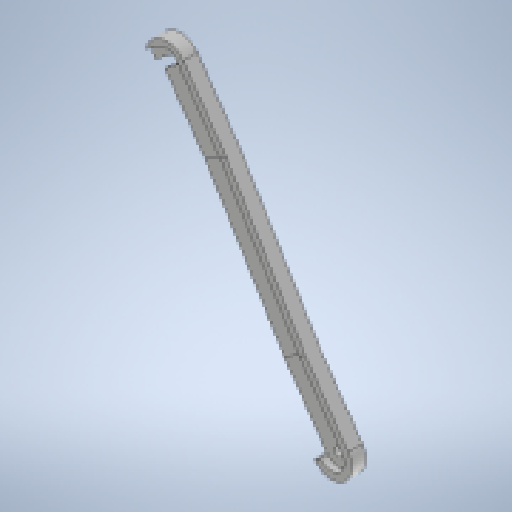
# Autodesk Inventor part: TheHandle_LeftBack
Saved by Autodesk Inventor 2025.1 (Build 291241000, 241)
## iProperties
Created: 2026-05-10
Part Number: TheHandle_LeftBack
Material: Generic
Document SubType Name: Modeling
Designer: User
Density: 1 g/cm^3
Appearance: Default
Author: User
## iProperties of the stored document TheHandle_LeftBack_3DPrint.ipt
Created: 2026-05-12
Part Number: TheHandle_LeftBack_3DPrint
Material: Generic
Document SubType Name: Modeling
Designer: User
Density: 1 g/cm^3
Appearance: Default
Author: User
Autodesk Inventor part; units mm, degrees
ref_plane "YZ Plane" through (0, 0, 0) normal (1, 0, 0) x (0, 1, 0)
ref_plane "XZ Plane" through (0, 0, 0) normal (0, 1, 0) x (-1, 0, 0)
ref_plane "XY Plane" through (0, 0, 0) normal (0, 0, 1) x (1, 0, 0)
sketch "Sketch1" plane through (0, 0, 0) normal (0, 0, 1) x (1, 0, 0)
  arc A0 (17.8, -18.3349) -> (28.2, -18.3349) centre (23, -18.3349) ccw projected
  circle A1 centre (120.0032, -158.8554) radius 2.5 projected
  arc A2 (212.7339, -15.835) -> (209.4702, -20.8697) centre (211.0753, -18.3349) ccw projected
  circle A3 centre (23, -18.3349) radius 2.5
  circle A4 centre (23, -18.3349) radius 7.5
  circle A5 centre (120.0032, -158.8554) radius 7.5
  line L0 (113.831, -163.1162) -> (16.8278, -22.5957)
  line L1 (126.1754, -154.5947) -> (29.1722, -14.0742)
  point P0 (0, 0)
  dimension "d0" = 5
  dimension "d1" = 15
  dimension "d2" = 15
  constraints: 4 end point, 4 point on circle, 4 tangent, 3 centre point, 3 coincident
  measures "d0" diameter of A3
  measures "d1" diameter of A4
  measures "d2" diameter of A5
extrude "Extrusion1" add sketch "Sketch1" along normal blind 4
sketch "Sketch2" plane through (113.831, -163.1162, 0) normal (-0.8229595, -0.5681, 0) x (0, 0, 1)
  line L0 (4, 170.7502) -> (4, 0) projected
  line L1 (8, 170.7502) -> (8, 0)
  line L2 (8, 85.3751) -> (0, 85.3751)
  line L3 (0, 170.7502) -> (0, 0) projected
  line L4 (8, 0) -> (8, 85.3751)
  line L5 (8, 42.6875) -> (0, 42.6875)
  line L6 (8, 170.7502) -> (8, 85.3751)
  line L7 (8, 128.0626) -> (0, 128.0626)
  line L8 (4, 42.6875) -> (0, 128.0626)
  line L9 (8, 42.6875) -> (4, 128.0626)
  line L10 (8, 0) -> (4, 0)
  point P0 (0, 198.9054)
  dimension "d5" = 4
  constraints: 18 end point, 6 midpoint, 3 perpendicular, 2 collinear, 2 point on line, 1 parallel
  measures "d5" distance between parallel lines of L0 L1
extrude "Extrusion2" add sketch "Sketch2" against normal up to surface (15 mm away) contours L5 L1 L10 L0 | L0 L2 L9 L5 | L0 L9 L2
sketch "Sketch3" plane through (16.8278, -22.5957, 0) normal (-0.8229595, -0.5681, 0) x (0, 0, 1)
  line L0 (0, 0) -> (0, -170.7502) projected
  line L1 (0, -170.7502) -> (4, -170.7502) projected
  line L2 (4, -170.7502) -> (8, -170.7502) projected
  line L3 (8, -170.7502) -> (8, -128.0626) projected
  line L4 (8, -128.0626) -> (4, -42.6875) projected
  line L5 (4, 0) -> (4, -42.6875) projected
  line L6 (0, 0) -> (4, 0) projected
  line L7 (4, -170.7502) -> (4, -173.2502) projected
  line L8 (4, -170.7502) -> (4, -42.6875)
  line L9 (0, -170.7502) -> (0, 0) projected
  line L10 (8, -170.7502) -> (8, -128.0626) projected
  line L11 (8, -128.0626) -> (4, -128.0626)
  line L12 (4, -128.0626) -> (0, -42.6875)
  line L13 (0, -178.2502) -> (4, -178.2502)
  line L14 (4, -166.4894) -> (4, -164.4356) projected
  line L15 (0, -178.2502) -> (0, -163.8178) projected
  point P0 (0, 28.1552)
  constraints: 6 end point, 2 parallel, 2 point on line, 1 perpendicular, 5 other
extrude "Extrusion3" cut sketch "Sketch3" against normal through all contours L12 L8 L1 L0 | L8 L4 L11
sketch "Sketch4" plane through (113.831, -163.1162, 8) normal (0, 0, 1) x (0.8229595, 0.5681, 0)
  circle A0 centre (7.5, 0) radius 2.5 projected
  arc A1 (3.4533, 6.3146) -> (1.3278, 4.2607) centre (7.5, 0) ccw projected
  circle A2 centre (7.5, 0) radius 2.5
  point P0 (-1.012, 198.9054)
  constraints: 1 centre point, 1 coincident, 1 concentric
extrude "Extrusion4" cut sketch "Sketch4" against normal blind 10
sketch "Sketch5" plane through (113.831, -163.1162, 8) normal (0, 0, 1) x (0.8229595, 0.5681, 0)
  circle A0 centre (7.5, 0) radius 2.5 projected
  line L0 (15, 0) -> (15, 42.6875) projected
  line L1 (0, 0) -> (0, 42.6875) projected
  line L2 (10, 0) -> (15, 0) projected
  circle A1 centre (7.5, 0) radius 7.5
  point P0 (-1.012, 198.9054)
  constraints: 2 horizontal alignment, 1 coincident, 2 other
extrude "Extrusion5" add sketch "Sketch5" against normal blind 4
sketch "Sketch6" plane through (0, 0, 4) normal (0, 0, 1) x (1, 0, 0)
  circle A0 centre (23, -18.3349) radius 2.5 projected
  line L0 (53.423, -49.2043) -> (29.1722, -14.0742) projected
  arc A1 (18.7282, -24.4995) -> (16.8278, -22.5957) centre (23, -18.3349) ccw
  circle A2 centre (120.0032, -158.8554) radius 2.5 projected
  arc A3 (24.4203, -20.3923) -> (18.3431, -24.7907) centre (120.0032, -158.8554) ccw
  arc A4 (21.5797, -16.2775) -> (15.8025, -20.4436) centre (120.0032, -158.8554) ccw
  line L1 (16.8278, -22.5957) -> (41.0786, -57.7258) projected
  point P0 (0, 0)
  dimension "d14" = 5
  constraints: 11 point on circle, 3 centre point, 2 coincident, 1 end point, 1 point on line, 1 tangent
  measures "d14" radial gap between concentric circles of A3 A4
extrude "Extrusion6" cut sketch "Sketch6" against normal blind 4 contours A0 A3 L1 A1 A4
sketch "Sketch7" plane through (29.1722, -14.0742, 4) normal (0.8229595, 0.5681, 0) x (0, 0, -1)
  line L0 (0, -128.0626) -> (4, -42.6875) projected
  line L1 (4, -42.6875) -> (4, 0) projected
  line L2 (4, 0) -> (0, 0) projected
  line L3 (0, -128.0626) -> (0, 0) projected
  line L4 (-4, -170.7502) -> (-4, -128.0626) projected
  line L5 (1.4491, -170.7502) -> (-4, -170.7502) projected
  line L6 (0, -166.4894) -> (0, -128.0626) projected
  line L7 (-8, -127.969) -> (-4, -42.5939)
  line L8 (-4, -42.5939) -> (-4, 4)
  line L9 (-4, 4) -> (8, 4)
  line L10 (8, 4) -> (8, -42.7812)
  line L11 (8, -42.7812) -> (4, -128.1563)
  line L12 (4, -128.1563) -> (4, -174.7502)
  line L13 (4, -174.7502) -> (-8, -174.7502)
  line L14 (-8, -174.7502) -> (-8, -127.969)
  line L15 (-8, -170.7502) -> (0, -170.7502)
  line L16 (-4, 0) -> (4, 0)
  line L17 (1.4491, -170.7502) -> (0, -166.4894) projected
  line L18 (0, -128.0626) -> (-4, -128.0626) projected
  point P0 (4, 28.1552)
  point P1 (-4, -170.7502)
  point P2 (0, 0)
  point P3 (-4, -170.7502)
  dimension "d17" = 4
  constraints: 20 end point, 2 point on line, 1 collinear, 1 perpendicular, 6 other
  measures "d17" distance between parallel lines of L4 L14
extrude "Extrusion7" add sketch "Sketch7" along normal blind 4
sketch "Sketch8" plane through (0, 0, 0) normal (0, 0, -1) x (-1, 0, 0)
  arc A0 (-15.8025, -20.4436) -> (-29.1722, -14.0742) centre (-23, -18.3349) ccw
  arc A1 (-15.8025, -20.4436) -> (-21.5797, -16.2775) centre (-120.0032, -158.8554) ccw projected
  arc A2 (-14.7318, -26.3279) -> (-32.464, -11.8018) centre (-23, -18.3349) ccw
  arc A3 (-14.7318, -26.3279) -> (-23.8522, -19.5694) centre (-120.0032, -158.8554) ccw
  line L0 (-21.5797, -16.2775) -> (-15.8025, -20.4436)
  line L1 (-21.5797, -16.2775) -> (-12.4333, -22.8731)
  line L2 (-29.1722, -14.0742) -> (-32.464, -11.8018)
  point P0 (0, 0)
  point P1 (-15.8025, -20.4436)
  dimension "d20" = 4
  constraints: 7 point on circle, 6 end point, 3 centre point, 1 point on line
  measures "d20" radial gap between concentric circles of A0 A2
extrude "Extrusion8" add sketch "Sketch8" against normal up to surface (8 mm away) contours A0 L2 A2 L1
sketch "Sketch9" plane through (56.6616, -46.8548, 8) normal (0, 0, 1) x (0.8229595, 0.5681, 0)
  arc A0 (-0.7181, 46.5939) -> (-22.7741, 44.8621) centre (-11.5, 42.5939) ccw projected
  line L0 (0, 46.5939) -> (0, 0) projected
  circle A1 centre (-11.5, 42.5939) radius 11.5
  line L1 (-0.7181, 46.5939) -> (0, 46.5939) projected
  point P0 (-20.012, 70.7491)
  point P1 (-0.7181, 46.5939)
  point P2 (0, 42.5939)
  constraints: 1 centre point, 1 coincident, 1 tangent
extrude "Extrusion9" cut sketch "Sketch9" against normal through all contours L1 L0 A1
sketch "Sketch10" plane through (18.3431, -24.7907, 0) normal (-0.8229595, -0.5681, 0) x (0, 0, 1)
  line L0 (0, -40.0203) -> (4, -125.3954) projected
  line L1 (8, -125.3954) -> (4, -125.3954) projected
  line L2 (4, 0) -> (4, -125.3954) projected
  line L3 (0, -40.0203) -> (4, -40.0203)
  line L4 (0, -40.0203) -> (4, -40.0203) construction
  line L5 (8, -125.3954) -> (4, -40.0203)
  point P0 (0, 30.8225)
  dimension "d25" = 0
  constraints: 6 end point, 1 collinear, 1 horizontal, 1 point on line
  measures "d25" distance between parallel lines of L3 L4
extrude "Extrusion10" add sketch "Sketch10" against normal blind 15 contours L2 L5 L1
sketch "Sketch11" plane through (113.831, -163.1162, 2.5509) normal (-0.8229595, -0.5681, 0) x (0, 0, 1)
  line L0 (5.4491, -7.5) -> (5.4491, 0) projected
  line L1 (5.4491, 0) -> (5.4491, 42.6875) projected
  line L2 (5.4491, 42.6875) -> (1.4491, 128.0626) projected
  line L3 (1.4491, 168.0829) -> (1.4491, 128.0626) projected
  line L4 (1.4491, 173.2502) -> (1.4491, 168.2502) projected
  line L5 (-2.5509, 173.0184) -> (-2.5509, 174.7502) projected
  line L6 (-2.5509, 173.0184) -> (5.4491, 173.0184) projected
  line L7 (5.4491, 170.7502) -> (5.4491, 173.0184) projected
  line L8 (-6.5509, 170.7502) -> (5.4491, 170.7502) projected
  line L9 (-6.5509, 174.7502) -> (-6.5509, 170.7502) projected
  line L10 (-2.5509, 174.7502) -> (-6.5509, 174.7502) projected
  line L11 (5.4491, 170.7502) -> (5.4491, 128.1563) projected
  line L12 (5.4491, 128.1563) -> (9.4491, 42.7812) projected
  line L13 (9.4491, 42.7812) -> (9.4491, -4) projected
  line L14 (9.4491, -4) -> (-2.5509, -4) projected
  line L15 (5.4491, 170.7502) -> (5.4491, 182.2502) projected
  line L16 (-2.5509, 182.2502) -> (5.4491, 182.2502) projected
  line L17 (5.4491, 170.7502) -> (1.4491, 170.7502)
  line L18 (1.4491, 170.7502) -> (1.4491, 182.2502)
  line L19 (1.4491, 182.2502) -> (5.4491, 182.2502)
  line L20 (5.4491, 182.2502) -> (5.4491, 170.7502)
  line L21 (1.4491, 128.0626) -> (5.4491, 42.6875) projected
  line L22 (5.4491, 0) -> (5.4491, 42.6875) projected
  line L23 (0, 0) -> (5.4491, 0) projected
  line L24 (0, 0) -> (1.4491, 4.2607) projected
  line L25 (1.4491, 4.2607) -> (1.4491, 42.6875) projected
  line L26 (1.4491, 42.6875) -> (-2.5509, 128.0626) projected
  line L27 (-2.5509, 128.0626) -> (-2.5509, 174.7502) projected
  line L28 (-6.5509, 174.7502) -> (-2.5509, 174.7502) projected
  line L29 (-6.5509, 127.969) -> (-6.5509, 174.7502) projected
  line L30 (-2.5509, 42.5939) -> (-6.5509, 127.969) projected
  line L31 (-2.5509, -4) -> (-2.5509, 42.5939) projected
  line L32 (9.4491, -4) -> (-2.5509, -4) projected
  line L33 (9.4491, 42.7812) -> (9.4491, -4) projected
  line L34 (5.4491, 128.1563) -> (9.4491, 42.7812) projected
  line L35 (5.4491, 170.7502) -> (5.4491, 128.1563) projected
  line L36 (5.4491, 170.7502) -> (1.4491, 170.7502) projected
  line L37 (1.4491, 128.0626) -> (1.4491, 170.7502) projected
  line L38 (1.4491, 4.2607) -> (1.4491, -4)
  line L39 (1.4491, 128.0626) -> (5.4491, 42.6875) projected
  line L40 (5.4491, 0) -> (5.4491, 42.6875) projected
  line L41 (0, 0) -> (5.4491, 0) projected
  line L42 (0, 0) -> (1.4491, 4.2607) projected
  line L43 (1.4491, 4.2607) -> (1.4491, 42.6875) projected
  line L44 (1.4491, 42.6875) -> (-2.5509, 128.0626) projected
  line L45 (-2.5509, 128.0626) -> (-2.5509, 174.7502) projected
  line L46 (-6.5509, 174.7502) -> (-2.5509, 174.7502) projected
  line L47 (-6.5509, 127.969) -> (-6.5509, 174.7502) projected
  line L48 (-2.5509, 42.5939) -> (-6.5509, 127.969) projected
  line L49 (-2.5509, -4) -> (-2.5509, 42.5939) projected
  line L50 (9.4491, -4) -> (-2.5509, -4) projected
  line L51 (9.4491, 42.7812) -> (9.4491, -4) projected
  line L52 (5.4491, 128.1563) -> (9.4491, 42.7812) projected
  line L53 (5.4491, 170.7502) -> (5.4491, 128.1563) projected
  line L54 (5.4491, 170.7502) -> (1.4491, 170.7502) projected
  line L55 (1.4491, 128.0626) -> (1.4491, 170.7502) projected
  line L56 (-6.5509, 127.969) -> (-6.5509, 174.7502) projected
  line L57 (-6.5509, 174.7502) -> (-2.5509, 174.7502) projected
  line L58 (-2.5509, 182.2502) -> (-2.5509, 173.0184) projected
  line L59 (-2.5509, 174.7502) -> (-6.5509, 174.7502) projected
  line L60 (1.4491, 4.2607) -> (1.4491, -4)
  point P0 (-2.5509, 198.9054)
  point P1 (-2.5509, 173.0184)
  point P2 (-2.5509, -4)
  point P3 (1.4491, -4)
  constraints: 12 end point, 2 parallel, 2 vertical, 1 horizontal, 1 midpoint, 1 perpendicular, 1 point on line
extrude "Extrusion11" cut sketch "Sketch11" against normal blind 147.359 contours L14 L31 L30 L29 L8 L27 L26 L25 L24 L23 L38 | L23 L24 L38 | L9 L10 L5 L27 L8
sketch "Sketch12" plane through (113.831, -163.1162, 4) normal (-0.8229595, -0.5681, 0) x (0, 0, 1)
  line L0 (0, 42.6875) -> (0, 0) projected
  line L1 (0, 0) -> (-8.279, 0)
  line L2 (-8.279, 0) -> (-8.279, -22.088)
  line L3 (-8.279, -22.088) -> (0, -22.088)
  line L4 (0, -22.088) -> (0, 0)
  point P0 (-4, 198.9054)
  constraints: 8 end point, 2 parallel, 1 horizontal, 1 perpendicular
extrude "Extrusion12" cut sketch "Sketch12" against normal blind 147.359
sketch "Sketch13" plane through (120.0032, -158.8554, 8) normal (0, 0, 1) x (0.8229595, 0.5681, 0)
  arc A0 (-7.5, 0) -> (7.5, 0) centre (0, 0) ccw projected
  arc A1 (-11.5, 0) -> (11.5, 0) centre (0, 0) ccw
  line L0 (11.5, 42.7812) -> (11.5, -4) projected
  line L1 (7.5, -4) -> (11.5, -4) projected
  line L2 (7.5, 42.7812) -> (7.5, -4) projected
  line L3 (-11.5, 0) -> (-7.5, 0)
  line L4 (7.5, 0) -> (11.5, 0)
  point P0 (-8.512, 198.9054)
  point P1 (10.7819, -4)
  dimension "d32" = 4
  constraints: 4 end point, 2 horizontal, 2 point on circle, 1 centre point
  measures "d32" radial gap between concentric circles of A0 A1
extrude "Extrusion13" cut sketch "Sketch13" along normal mid plane 147.359
sketch "Sketch14" plane through (113.831, -163.1162, 8) normal (0, 0, 1) x (0.8229595, 0.5681, 0)
  arc A0 (0, 0) -> (15, 0) centre (7.5, 0) ccw projected
  arc A1 (-4, 0) -> (19, 0) centre (7.5, 0) ccw
  line L0 (-4, 0) -> (0, 0)
  line L1 (15, 0) -> (19, 0)
  point P0 (-1.012, 198.9054)
  dimension "d35" = 4
  constraints: 4 end point, 2 point on circle, 1 centre point, 1 collinear, 1 horizontal
  measures "d35" radial gap between concentric circles of A0 A1
extrude "Extrusion14" add sketch "Sketch14" along normal mid plane 8
sketch "Sketch15" plane through (53.3698, -49.1272, 8) normal (0, 0, 1) x (0.8229595, 0.5681, 0)
  arc A0 (0, 42.5939) -> (-14.6211, 44.9475) centre (-7.5, 42.5939) ccw projected
  line L0 (0, 42.5939) -> (0, 0) projected
  line L1 (0.5, 0) -> (0.5, 42.5939)
  arc A1 (0.5, 42.5939) -> (-15.0959, 45.1044) centre (-7.5, 42.5939) ccw
  arc A2 (-7.5, 40.0939) -> (-7.5, 45.0939) centre (-7.5, 42.5939) ccw projected
  circle A3 centre (-7.5, 42.5939) radius 8
  line L2 (-7.5, 42.5939) -> (-7.5, 54.0939)
  arc A4 (4, 42.5939) -> (-18.7741, 44.8621) centre (-7.5, 42.5939) ccw projected
  line L3 (-7.5, 50.5939) -> (-18.4679, 50.5939)
  line L4 (-14.6211, 44.9475) -> (-18.7741, 44.8621) projected
  point P0 (-16.012, 70.7491)
  point P1 (0, 39.81)
  point P2 (-7.5, 50.5939)
  point P3 (-15.7614, 50.5939)
  dimension "d38" = 0.5
  constraints: 6 end point, 5 point on circle, 2 centre point, 2 tangent, 1 coincident, 1 perpendicular, 1 point on line, 1 vertical, 1 other
  measures "d38" distance between parallel lines of L0 L1
extrude "Extrusion15" cut sketch "Sketch15" against normal up to surface (4 mm away) contours A0 L2 A1 A3 L0 | A0 L4 A3 A1 L2 | A1 A3 L4 A4 L3
sketch "Sketch16" plane through (89.5802, -127.986, 8) normal (-0.0265875, 0.0385151, 0.9989042) x (0.8229595, 0.5681, 0)
  line L0 (3.2634, 69.5858) -> (3.2634, 85.4325) construction
  line L1 (3.2634, 85.4325) -> (12.4226, 85.4325) construction
  line L2 (12.4226, 85.4325) -> (12.4226, 69.5858) construction
  line L3 (12.4226, 69.5858) -> (3.2634, 69.5858) construction
  line L4 (12.4226, 76.6444) -> (12.4226, 70.5359)
  line L5 (12.4226, 70.5359) -> (3.2634, 70.5359)
  line L6 (3.2634, 70.5359) -> (3.2634, 72.8368)
  line L7 (3.2634, 72.8368) -> (10.6783, 72.8368)
  line L8 (10.6783, 72.8368) -> (10.6783, 76.6444)
  line L9 (10.6783, 76.6444) -> (12.4226, 76.6444)
  spline S0 degree 2 poles (9.6169, 85.0614) (10.2998, 85.0614) (11.3315, 84.5418) (11.6729, 84.1113) knots 0 0 0 1 2 2 2
  spline S1 degree 2 poles (11.6729, 84.1113) (12.0811, 83.5917) (12.4226, 82.3596) (12.4226, 81.4021) knots 0 0 0 1 2 2 2
  line L10 (12.4226, 81.4021) -> (12.4226, 77.7429)
  line L11 (12.4226, 77.7429) -> (3.2634, 77.7429)
  line L12 (3.2634, 77.7429) -> (3.2634, 80.9717)
  spline S2 degree 2 poles (3.2634, 80.9717) (3.2634, 81.9811) (3.4193, 83.0202) (3.6642, 83.473) knots 0 0 0 1 2 2 2
  spline S3 degree 2 poles (3.6642, 83.473) (3.924, 83.9703) (4.8147, 84.4527) (5.3936, 84.4527) knots 0 0 0 1 2 2 2
  spline S4 degree 2 poles (5.3936, 84.4527) (6.0616, 84.4527) (7.1082, 83.7847) (7.3531, 83.1909) knots 0 0 0 1 2 2 2
  line L13 (7.3531, 83.1909) -> (7.3976, 83.1909)
  spline S5 degree 2 poles (7.3976, 83.1909) (7.5758, 84.0445) (8.6817, 85.0614) (9.6169, 85.0614) knots 0 0 0 1 2 2 2
  spline S6 degree 2 poles (9.5798, 82.6862) (9.1493, 82.6862) (8.6669, 82.3448) (8.5407, 82.0034) knots 0 0 0 1 2 2 2
  spline S7 degree 2 poles (8.5407, 82.0034) (8.459, 81.7955) (8.4442, 81.0607) (8.4442, 80.4521) knots 0 0 0 1 2 2 2
  line L14 (8.4442, 80.4521) -> (8.4442, 80.029)
  line L15 (8.4442, 80.029) -> (10.7525, 80.029)
  line L16 (10.7525, 80.029) -> (10.7525, 80.1552)
  spline S8 degree 2 poles (10.7525, 80.1552) (10.7525, 81.0459) (10.7303, 81.7287) (10.5744, 82.085) knots 0 0 0 1 2 2 2
  spline S9 degree 2 poles (10.5744, 82.085) (10.4334, 82.3967) (9.9138, 82.6862) (9.5798, 82.6862) knots 0 0 0 1 2 2 2
  spline S10 degree 2 poles (5.8464, 82.1147) (5.6237, 82.1147) (5.1561, 81.8846) (5.0522, 81.6471) knots 0 0 0 1 2 2 2
  spline S11 degree 2 poles (5.0522, 81.6471) (4.9483, 81.4244) (4.9334, 80.8009) (4.9334, 80.1849) knots 0 0 0 1 2 2 2
  line L17 (4.9334, 80.1849) -> (4.9334, 80.029)
  line L18 (4.9334, 80.029) -> (6.8781, 80.029)
  line L19 (6.8781, 80.029) -> (6.8781, 80.3185)
  spline S12 degree 2 poles (6.8781, 80.3185) (6.8781, 80.9049) (6.8558, 81.3799) (6.7371, 81.6322) knots 0 0 0 1 2 2 2
  spline S13 degree 2 poles (6.7371, 81.6322) (6.6035, 81.9069) (6.1507, 82.1147) (5.8464, 82.1147) knots 0 0 0 1 2 2 2
  point P0 (-1.012, 156.4211)
  constraints: 2 other
emboss "Emboss1" sketch "Sketch16" operation cut depth 0.5 direction (0.0265875, -0.0385151, -0.9989042)
body "Solid1"
